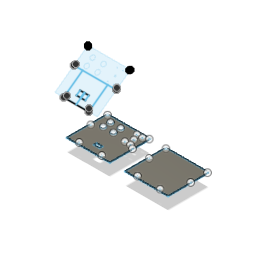
prop-blueprint (Autodesk Fusion 360 archive; units mm, degrees)
design "ledmatrix"
Autodesk Fusion 360 part; units mm, degrees
sketch "Sketch1" plane through (0, 0, 0) normal (0, 1, 0) x (1, 0, 0)
  line L0 (0, 0) -> (192, 0)
  line L1 (192, 0) -> (192, -96)
  line L2 (192, -96) -> (0, -96)
  line L3 (0, -96) -> (0, 0)
  line L4 (0, 0) -> (12, 0)
  line L5 (0, 0) -> (0, -10)
  line L6 (0, -10) -> (20.9444, -10)
  line L7 (12, 0) -> (12, -10)
  circle A0 centre (12, -10) radius 1.5
  circle A1 centre (113.3925, -144.8414) radius 15
  line L8 (283.7254, -24.5165) -> (335.7254, -24.5165)
  line L9 (335.7254, -24.5165) -> (335.7254, -119.5165)
  line L10 (335.7254, -119.5165) -> (283.7254, -119.5165)
  line L11 (283.7254, -119.5165) -> (283.7254, -24.5165)
  line L12 (283.7254, -24.5165) -> (290.7254, -24.5165)
  line L13 (290.7254, -24.5165) -> (290.7254, -30.5165)
  circle A2 centre (290.7254, -30.5165) radius 2.5
  dimension "d1" = 192
  dimension "d2" = 96
  dimension "d3" = 12
  dimension "d4" = 10
  dimension "d5" = 3
  dimension "d6" = 30
  dimension "d7" = 52
  dimension "d8" = 95
  dimension "d9" = 7
  dimension "d10" = 6
  dimension "d11" = 5
  constraint horizontal L0
  constraint vertical L1
  constraint horizontal L2
  constraint vertical L3
  constraint coincident L0.start L3.end
  constraint perpendicular L3 L4
  constraint perpendicular L4 L5
  constraint perpendicular L3 L6
  constraint coincident L6 L7.end
  constraint perpendicular L6 L7
  constraint coincident L7.end A0.centre
  constraint horizontal L8
  constraint vertical L9
  constraint horizontal L10
  constraint vertical L11
  constraint perpendicular L11 L12
  constraint perpendicular L12 L13
  constraint coincident L13.end A2.centre
  measures "d1" distance of L0.start L0.end
  measures "d2" distance of L0.start L2.end
  measures "d3" distance of L0.start L4.end
  measures "d4" distance of L0.start L5.end
  measures "d5" diameter of A0
  measures "d6" diameter of A1
  measures "d7" distance of L8.start L8.end
  measures "d8" distance of L8.start L10.end
  measures "d9" distance of L8.start L12.end
  measures "d10" distance of L12.end L13.end
  measures "d11" diameter of A2
sketch "Sketch2" plane through (96, 0, 48) normal (0, 1, 0) x (1, 0, 0)
  line L0 (-96, -48) -> (96, -48)
  line L1 (96, -48) -> (96, -58)
  line L2 (96, -58) -> (-96, -58)
  line L3 (-96, -58) -> (-96, -48)
  line L4 (-96, -58) -> (-116, -58)
  line L5 (-116, -58) -> (-116, 48)
  line L6 (-116, 48) -> (-96, 48)
  line L7 (-96, 48) -> (-96, -58)
  line L8 (96, -58) -> (116, -58)
  line L9 (116, -58) -> (116, 48)
  line L10 (116, 48) -> (96, 48)
  line L11 (96, 48) -> (96, -58)
  line L12 (-116, 48) -> (116, 48)
  line L13 (116, 48) -> (116, 58)
  line L14 (116, 58) -> (-116, 58)
  line L15 (-116, 58) -> (-116, 48)
  line L16 (-96, 38) -> (96, 38)
  line L17 (-84, 48) -> (-84, -48)
  line L18 (-96, -48) -> (-96, -38)
  line L19 (-96, -38) -> (96, -38)
  line L20 (96, -48) -> (84, -48)
  line L21 (96, -48) -> (84, -48)
  line L22 (84, -48) -> (84, 48)
  dimension "d12" = 10
  dimension "d13" = 20
  dimension "d14" = 20
  dimension "d15" = 10
  dimension "d16" = 192
  dimension "d17" = 96
  constraint horizontal L0
  constraint vertical L1
  constraint horizontal L2
  constraint vertical L3
  constraint horizontal L4
  constraint vertical L5
  constraint horizontal L6
  constraint vertical L7
  constraint horizontal L8
  constraint vertical L9
  constraint horizontal L10
  constraint vertical L11
  constraint horizontal L12
  constraint vertical L13
  constraint horizontal L14
  constraint vertical L15
  constraint coincident L7 L16.start
  constraint coincident L11 L16.end
  constraint perpendicular L11 L16
  constraint coincident L12 L17.start
  constraint coincident L0 L17.end
  constraint perpendicular L0 L17
  constraint coincident L7 L18.end
  constraint coincident L11 L19.end
  constraint perpendicular L11 L19
  constraint coincident L0 L20.end
  constraint coincident L12 L22.end
  constraint perpendicular L12 L22
  measures "d12" distance of L0.start L2.end
  measures "d13" distance of L2.end L4.end
  measures "d14" distance of L1.end L8.end
  measures "d15" distance of L5.end L14.end
  measures "d16" distance of L18.end L19.end
  measures "d17" distance of L17.start L17.end
extrude "Extrude1" add sketch "Sketch2" along normal blind 10 contours L0 L1 L2 L3 L7 L11 L20 L21 | L3 L4 L5 L6 L7 L12 L18 | L1 L8 L9 L10 L11 L12 | L6 L10 L12 L13 L14 L15 makes body 1
extrude "Extrude2" add sketch "Sketch2" against normal blind 10 contours L0 L7 L17 L18 L19 | L0 L1 L2 L3 L7 L11 L20 L21 | L3 L4 L5 L6 L7 L12 L18 | L0 L17 L19 L22 | L7 L16 L17 L19 | L0 L11 L19 L20 L21 L22 | L1 L8 L9 L10 L11 L12 | L7 L12 L16 L17 | L11 L16 L19 L22 | L12 L16 L17 L22 | L6 L10 L12 L13 L14 L15 | L11 L12 L16 L22 bodies 1
move_body "Move1" bodies 1 to x (1, 0, 0) y (0, 1, 0) z (0, 0, 1) at (260, 0, 0)
sketch "Sketch3" plane through (0, 0, 0) normal (0, 1, 0) x (1, 0, 0)
  line L0 (0, 0) -> (0, 136)
  line L1 (0, 0) -> (64.6952, 47.0588)
  line L2 (64.6952, 47.0588) -> (0, 136)
  dimension "d22" = 136
  dimension "d23" = 80
  constraint vertical L0
  measures "d22" distance of L0.start L0.end
  measures "d23" distance of L0.start L1.end
sketch "Sketch4" plane through (240, 0, 0) normal (-1, 0, 0) x (0, 0, 1)
  line L0 (106, -10) -> (106, 10)
  line L1 (106, 10) -> (-10, 10)
  line L2 (-10, 10) -> (-10, -10)
  line L3 (-10, -10) -> (106, -10)
  line L4 (-50, 10) -> (70.9677, -78.695)
  line L5 (70.9677, -78.695) -> (80.0728, -85.371)
  line L6 (150, 10) -> (80.0728, -85.371)
  line L7 (150, 10) -> (-50, 10)
  dimension "d27" = 150
  constraint perpendicular L5 L6
  constraint parallel L1 L7
  measures "d27" distance of L4.start L4.end
extrude "Extrude4" add sketch "Sketch4" along normal blind 30 separate body makes body 2
sketch "Sketch5" plane through (502, 0, 0) normal (1, 0, 0) x (0, 0, -1)
  line L0 (-80.0728, -85.371) -> (50, 10)
  line L1 (50, 10) -> (-150, 10)
  line L2 (-80.0728, -85.371) -> (-77.1163, -89.4032)
  line L3 (149.7307, 76.9238) -> (146.7742, 80.956)
  line L4 (-150, 10) -> (-80.0728, -85.371)
  line L5 (-80.0728, -85.371) -> (146.7742, 80.956)
  line L6 (149.7307, 76.9238) -> (-77.1163, -89.4032)
  dimension "d58" = 5
  constraint coincident L0.start L2.start
  constraint perpendicular L3 L5
  constraint perpendicular L2 L6
  measures "d58" distance of L3.end L3.start
move_body "Move6" bodies 1 to x (1, 0, 0) y (0, 1, 0) z (0, 0, 1) at (0, 0, -2.5)
sketch "Sketch6" plane through (472, 0, 0) normal (1, 0, 0) x (0, 0, -1)
  line L0 (12.5, -10) -> (12.5, 10)
  line L1 (12.5, 10) -> (-103.5, 10)
  line L2 (-103.5, 10) -> (-103.5, -10)
  line L3 (-103.5, -10) -> (12.5, -10)
  line L4 (12.5, -10) -> (40, 10)
  line L5 (40, 10) -> (12.5, 10)
  constraint coincident L0.start L3.end
  constraint coincident L0.end L1.start
  constraint perpendicular L0 L5
extrude "Extrude6" add sketch "Sketch6" against normal blind 232 contours L0 L4 L5 bodies 1
sketch "Sketch7" plane through (0, -17.3391, -12.7132) normal (0, 0.806452, 0.5913) x (1, 0, 0)
  line L0 (502, -115.0547) -> (502, 166.2356)
  line L1 (502, 166.2356) -> (210, 166.2356)
  line L2 (210, 166.2356) -> (210, -115.0547)
  line L3 (210, -115.0547) -> (502, -115.0547)
  line L4 (270, -103.7625) -> (270, -90)
  line L5 (270, -90) -> (270, 46)
  line L6 (240, 46) -> (240, -103.7625)
  line L7 (240, 46) -> (240, 46.2347)
  line L8 (240, 46.2347) -> (270, 46.2347)
  line L9 (270, 46.2347) -> (270, 46)
  line L10 (240, -103.7625) -> (240, -115.0547)
  line L11 (270, -103.7625) -> (270, -115.0547)
  line L12 (240, -115.0547) -> (270, -115.0547)
  dimension "d40" = 30
  constraint perpendicular L7 L8
  constraint coincident L3 L10.end
  constraint perpendicular L3 L10
  constraint coincident L3 L11.end
  constraint perpendicular L3 L11
  measures "d40" distance of L6.end L4.start
extrude "Extrude7" add sketch "Sketch7" along normal blind 10 contours L3 L4 L5 L6 L7 L8 L9 L10 L11 L12 bodies 2
sketch "Sketch8" plane through (240, 0, 0) normal (-1, 0, 0) x (0, 0, 1)
  line L0 (-49.7079, 10) -> (-33.0881, 10)
  line L1 (-33.0881, 10) -> (-43.897, 17.9252)
  line L2 (-49.7079, 10) -> (-33.0881, 10)
  line L3 (-33.0881, 19.9922) -> (-49.7079, 19.9922)
  line L4 (-33.0881, 19.9922) -> (-33.0881, 10)
  line L5 (-43.897, 17.9252) -> (-49.7079, 10)
  line L6 (-49.7079, 10) -> (-50, 10)
  line L7 (-50, 10) -> (-50, 20)
  line L8 (-50, 20) -> (-49.7079, 19.9922)
  constraint coincident L0.start L2.start
  constraint coincident L0.end L1.start
  constraint parallel L0 L3
  constraint perpendicular L3 L4
  constraint perpendicular L2 L7
extrude "Extrude8" cut sketch "Sketch8" against normal blind 30 bodies 2
sketch "Sketch9" plane through (240, 0, 0) normal (1, 0, 0) x (0, 0, -1)
  line L0 (-85.9858, -77.3065) -> (33.0881, 10)
  line L1 (33.0881, 10) -> (-150, 10)
  line L2 (33.0881, 10) -> (33.0881, 0)
  line L3 (33.0881, 0) -> (3.0881, 0)
  line L4 (33.0881, 10) -> (3.0881, 10)
  line L5 (-150, 10) -> (-85.9858, -77.3065)
  line L6 (3.0881, 0) -> (-11.9119, 0)
  line L7 (3.0881, 10) -> (-11.9119, 0)
  dimension "d45" = 30
  dimension "d98" = 30
  dimension "d99" = 15
  constraint coincident L0.end L1.start
  constraint perpendicular L1 L2
  constraint perpendicular L2 L3
  constraint coincident L1 L4.end
  constraint parallel L3 L6
  measures "d45" distance of L2.end L3.end
  measures "d98" distance of L0.end L4.end
  measures "d99" distance of L3.end L6.end
extrude "Extrude9" add sketch "Sketch9" along normal blind 30 contours L0 L1 L3 L4 L6 L7 bodies 2
move_body "Move7" bodies 1 to x (1, 0, 0) y (0, 1, 0) z (0, 0, 1) at (0, -5, 15)
move_body "Move8" bodies 1 to x (1, 0, 0) y (0, 1, 0) z (0, 0, 1) at (0, -5, 6)
move_body "Move9" bodies 1 to x (1, 0, 0) y (0, 1, 0) z (0, 0, 1) at (0, 0, -0.5)
move_body "Move10" bodies 1 to x (1, 0, 0) y (0, 1, 0) z (0, 0, 1) at (0, 0, -0.1)
sketch "Sketch10" plane through (240, 0, 0) normal (1, 0, 0) x (0, 0, -1)
  line L0 (3.0881, 10) -> (-150, 10)
  line L1 (-150, 10) -> (-85.9858, -77.3065)
  line L2 (-85.9858, -77.3065) -> (19.4495, 0)
  line L3 (19.4495, 0) -> (-11.9119, 0)
  line L4 (-8.25, -20) -> (-8.25, -20.3096)
  line L5 (-8.25, -20.3096) -> (-68.25, -20.3096)
  line L6 (-68.25, -20.3096) -> (-68.25, -30.3096)
  line L7 (-8.25, -20.3096) -> (-21.8886, -30.3096)
  line L8 (-68.25, -30.3096) -> (-52.0404, -52.4173)
  line L9 (-124, 0) -> (-109, 0)
  line L10 (-109, 0) -> (-109, 10)
  line L11 (-109, 10) -> (-124, 10)
  line L12 (-124, 10) -> (-124, 0)
  line L13 (-11.9119, 0) -> (3.0881, 10)
  dimension "d50" = 10
  dimension "d51" = 60
  dimension "d91" = 15
  constraint coincident L2 L4.end
  constraint vertical L4
  constraint perpendicular L4 L5
  constraint perpendicular L5 L6
  constraint coincident L2 L7.end
  constraint coincident L2 L8.end
  constraint perpendicular L2 L8
  constraint horizontal L9
  constraint vertical L10
  constraint horizontal L11
  constraint vertical L12
  measures "d50" distance of L5.end L6.end
  measures "d51" distance of L4.end L5.end
  measures "d91" distance of L9.start L9.end
extrude "Extrude18" add sketch "Sketch10" along normal blind 30 contours L2 L5 L6 L7 L8 bodies 2
mirror "Mirror1" about plane through (0, 0, 0) normal (1, 0, 0) of bodies 2 makes body 3
sketch "Sketch11" plane through (0, -17.3391, -12.7132) normal (0, 0.806452, 0.5913) x (1, 0, 0)
  line L0 (502, -115.0547) -> (502, 166.2356)
  line L1 (502, 166.2356) -> (210, 166.2356)
  line L2 (210, 166.2356) -> (210, -115.0547)
  line L3 (210, -115.0547) -> (502, -115.0547)
  line L4 (475, 150) -> (423, 150)
  line L5 (423, 150) -> (423, 55)
  line L6 (423, 55) -> (475, 55)
  line L7 (475, 55) -> (475, 150)
  line L8 (423, 150) -> (430, 150)
  line L9 (430, 150) -> (430, 144)
  circle A0 centre (430, 144) radius 2.5
  line L10 (475, 150) -> (468, 150)
  line L11 (468, 150) -> (468, 144)
  circle A1 centre (468, 144) radius 2.5
  line L12 (475, 55) -> (468, 55)
  line L13 (468, 55) -> (468, 61)
  circle A2 centre (468, 61) radius 2.5
  line L14 (423, 55) -> (430, 55)
  line L15 (430, 55) -> (430, 61)
  circle A3 centre (430, 61) radius 2.5
  line L16 (423, 150) -> (449, 150)
  line L17 (449, 55) -> (449, 150)
  line L18 (475, 150) -> (475, 102.5)
  line L19 (475, 102.5) -> (423, 102.5)
  circle A4 centre (449, 102.5) radius 5
  dimension "d59" = 52
  dimension "d60" = 95
  dimension "d61" = 6
  dimension "d62" = 5
  dimension "d63" = 7
  dimension "d64" = 6
  dimension "d65" = 5
  dimension "d66" = 7
  dimension "d67" = 6
  dimension "d68" = 5
  dimension "d69" = 7
  dimension "d70" = 6
  dimension "d71" = 5
  dimension "d80" = 10
  constraint horizontal L4
  constraint vertical L5
  constraint horizontal L6
  constraint vertical L7
  constraint coincident L4 L8.end
  constraint perpendicular L4 L9
  constraint coincident L9.end A0.centre
  constraint perpendicular L7 L10
  constraint perpendicular L4 L11
  constraint coincident L11.end A1.centre
  constraint perpendicular L7 L12
  constraint perpendicular L12 L13
  constraint coincident L13.end A2.centre
  constraint perpendicular L5 L14
  constraint perpendicular L14 L15
  constraint coincident L15.end A3.centre
  constraint midpoint L4 L16.end
  constraint midpoint L6 L17.start
  constraint midpoint L7 L18.end
  constraint midpoint L5 L19.end
  constraint midpoint L19 A4.centre
  measures "d59" distance of L4.start L4.end
  measures "d60" distance of L4.start L6.end
  measures "d61" distance of L8.end L9.end
  measures "d62" diameter of A0
  measures "d63" distance of L4.start L10.end
  measures "d64" distance of L10.end L11.end
  measures "d65" diameter of A1
  measures "d66" distance of L6.end L12.end
  measures "d67" distance of L12.end L13.end
  measures "d68" diameter of A2
  measures "d69" distance of L5.end L14.end
  measures "d70" distance of L14.end L15.end
  measures "d71" diameter of A3
  measures "d80" diameter of A4
sketch "Sketch12" plane through (0, -17.3391, -12.7132) normal (0, 0.806452, 0.5913) x (1, 0, 0)
  circle A0 centre (275, 125) radius 15
  circle A1 centre (350, 125) radius 15
  circle A2 centre (275, 75) radius 15
  circle A3 centre (350, 75) radius 15
  dimension "d72" = 30
  dimension "d73" = 30
  dimension "d74" = 30
  dimension "d75" = 30
  measures "d72" diameter of A0
  measures "d73" diameter of A1
  measures "d74" diameter of A2
  measures "d75" diameter of A3
sketch "Sketch13" plane through (0, -21.3714, -15.6697) normal (0, -0.806452, -0.5913) x (-1, 0, 0)
  circle A0 centre (-430, 61) radius 2.5
  circle A1 centre (-468, 144) radius 2.5
  circle A2 centre (-468, 61) radius 2.5
  circle A3 centre (-430, 144) radius 2.5
  circle A4 centre (-449, 102.5) radius 5
  circle A5 centre (-350, 75) radius 15
  circle A6 centre (-350, 125) radius 15
  circle A7 centre (-275, 75) radius 15
  circle A8 centre (-275, 125) radius 15
  line L0 (-502, 166.2356) -> (-502, -115.0547)
  line L1 (-502, -115.0547) -> (-210, -115.0547)
  line L2 (-210, -115.0547) -> (-210, 166.2356)
  line L3 (-210, 166.2356) -> (-502, 166.2356)
  line L4 (-335, 125) -> (-290, 125)
  line L5 (-350, 110) -> (-350, 90)
  line L6 (-275, 110) -> (-275, 90)
  line L7 (-335, 75) -> (-290, 75)
  line L8 (-350, 100) -> (-275, 100)
  line L9 (-350, 100) -> (-361, 100)
  line L10 (-350, 100) -> (-355, 100)
  line L11 (-355, 100) -> (-355, 110.8579)
  line L12 (-350, 100) -> (-345, 100)
  line L13 (-345, 100) -> (-345, 110.8579)
  line L14 (-345, 100) -> (-345, 89.1421)
  line L15 (-355, 100) -> (-355, 89.1421)
  line L16 (-275, 100) -> (-270, 100)
  line L17 (-270, 100) -> (-270, 89.1421)
  line L18 (-270, 100) -> (-270, 110.8579)
  line L19 (-275, 100) -> (-280, 100)
  line L20 (-280, 100) -> (-280, 110.8579)
  line L21 (-280, 100) -> (-280, 89.1421)
  line L22 (-355, 89.1421) -> (-355, -115.0547)
  line L23 (-345, 89.1421) -> (-345, 80)
  line L24 (-345, 80) -> (-345, -115.0547)
  line L25 (-280, 89.1421) -> (-280, -115.0547)
  line L26 (-270, 89.1421) -> (-270, -115.0547)
  line L27 (-355, -115.0547) -> (-345, -115.0547)
  line L28 (-280, -115.0547) -> (-270, -115.0547)
  line L29 (-355, 110.8579) -> (-350, 110)
  line L30 (-345, 110.8579) -> (-350, 110)
  line L31 (-280, 110.8579) -> (-275, 110)
  line L32 (-270, 110.8579) -> (-275, 110)
  dimension "d81" = 5
  dimension "d82" = 5
  dimension "d83" = 10.8579
  constraint coincident A6 L4.start
  constraint coincident A8 L4.end
  constraint parallel L3 L4
  constraint coincident A6 L5.start
  constraint coincident A5 L5.end
  constraint perpendicular L4 L5
  constraint coincident A8 L6.start
  constraint coincident A7 L6.end
  constraint parallel L5 L6
  constraint coincident A5 L7.start
  constraint coincident A7 L7.end
  constraint perpendicular L6 L7
  constraint midpoint L5 L8.start
  constraint midpoint L6 L8.end
  constraint perpendicular L5 L9
  constraint coincident L9 L10.end
  constraint perpendicular L5 L10
  constraint coincident A6 L11.end
  constraint perpendicular L10 L11
  constraint coincident L8 L12.end
  constraint perpendicular L5 L12
  constraint coincident A6 L13.end
  constraint perpendicular L8 L13
  constraint coincident A5 L14.end
  constraint perpendicular L8 L14
  constraint coincident A5 L15.end
  constraint perpendicular L10 L15
  constraint perpendicular L6 L16
  constraint coincident A7 L17.end
  constraint perpendicular L8 L17
  constraint coincident A8 L18.end
  constraint perpendicular L16 L18
  constraint coincident L8 L19.end
  constraint perpendicular L6 L19
  constraint coincident A8 L20.end
  constraint perpendicular L19 L20
  constraint coincident A7 L21.end
  constraint perpendicular L8 L21
  constraint coincident L1 L22.end
  constraint perpendicular L1 L22
  constraint coincident L1 L24.end
  constraint perpendicular L1 L24
  constraint coincident L1 L25.end
  constraint perpendicular L1 L25
  constraint coincident L1 L26.end
  constraint perpendicular L1 L26
  measures "d81" distance of L8.end L19.end
  measures "d82" distance of L8.start L12.end
  measures "d83" distance of L12.end L13.end
extrude "Extrude15" cut 1 faces at (264, -10, 78.5667) along direction (0, -1, 0) blind 3 on bodies 1 bodies 1
fillet "Fillet1" radius 7.5 2 edges at (225, 10, 150) (-225, 10, 150) on bodies 2 3
move_body "Move15" bodies 3 to x (1, 0, 0) y (0, 1, 0) z (0, 0, 1) at (162, 0, 0)
sketch "Sketch15" plane through (0, -17.3391, -12.7132) normal (0, 0.806452, 0.5913) x (1, 0, 0)
  circle A0 centre (55, 61) radius 2.5
  circle A1 centre (93, 144) radius 2.5
  circle A2 centre (93, 61) radius 2.5
  circle A3 centre (55, 144) radius 2.5
  circle A4 centre (74, 102.5) radius 5
  circle A5 centre (-25, 75) radius 15
  circle A6 centre (-25, 125) radius 15
  circle A7 centre (-100, 75) radius 15
  circle A8 centre (-100, 125) radius 15
  line L0 (127, -115.0547) -> (127, 166.2356)
  line L1 (127, 166.2356) -> (-165, 166.2356)
  line L2 (-165, 166.2356) -> (-165, -115.0547)
  line L3 (-165, -115.0547) -> (127, -115.0547)
  line L4 (-165, 166.2356) -> (-160, 166.2356)
  line L5 (-160, 166.2356) -> (-160, 161.2356)
  line L6 (-160, 161.2356) -> (-165, 161.2356)
  line L7 (-165, 161.2356) -> (-165, 166.2356)
  circle A9 centre (-160, 161.2356) radius 1.5
  line L8 (127, 166.2356) -> (122, 166.2356)
  line L9 (122, 166.2356) -> (122, 161.2356)
  line L10 (122, 161.2356) -> (127, 161.2356)
  line L11 (127, 161.2356) -> (127, 166.2356)
  circle A10 centre (122, 161.2356) radius 1.5
  line L12 (-165, 46.3093) -> (-160, 46.3093)
  line L13 (-160, 46.3093) -> (-160, 56.3093)
  line L14 (-160, 56.3093) -> (-165, 56.3093)
  line L15 (-165, 56.3093) -> (-165, 46.3093)
  circle A11 centre (-160, 56.3093) radius 1.5
  line L16 (-160, 46.3093) -> (127, 46.3093)
  line L17 (127, 46.3093) -> (122, 46.3093)
  line L18 (122, 46.3093) -> (122, 56.3093)
  line L19 (122, 56.3093) -> (127, 56.3093)
  line L20 (127, 56.3093) -> (127, 46.3093)
  circle A12 centre (122, 56.3093) radius 1.5
  line L21 (-104.9331, 46.3093) -> (-104.9331, -115.0547)
  line L22 (67.0003, 46.3093) -> (67.0003, -115.0547)
  line L23 (67.0003, -115.0547) -> (57.0003, -115.0547)
  line L24 (57.0003, -115.0547) -> (57.0003, -100.0547)
  line L25 (57.0003, -100.0547) -> (67.0003, -100.0547)
  line L26 (67.0003, -100.0547) -> (67.0003, -115.0547)
  line L27 (-104.9331, -115.0547) -> (-94.9331, -115.0547)
  line L28 (-94.9331, -115.0547) -> (-94.9331, -100.0547)
  line L29 (-94.9331, -100.0547) -> (-104.9331, -100.0547)
  line L30 (-104.9331, -100.0547) -> (-104.9331, -115.0547)
  circle A13 centre (-94.9331, -100.0547) radius 1.5
  circle A14 centre (57.0003, -100.0547) radius 1.5
  line L31 (-104.9331, -115.0547) -> (67.0003, -115.0547)
  line L32 (-18.9664, -115.0547) -> (-18.9664, -45.0547)
  line L33 (-18.9664, -45.0547) -> (11.0336, -45.0547)
  line L34 (11.0336, -45.0547) -> (11.0336, -75.0547)
  line L35 (11.0336, -75.0547) -> (-18.9664, -75.0547)
  line L36 (-18.9664, -75.0547) -> (-18.9664, -45.0547)
  line L37 (-18.9664, -45.0547) -> (-48.9664, -45.0547)
  line L38 (-48.9664, -45.0547) -> (-48.9664, -75.0547)
  line L39 (-48.9664, -75.0547) -> (-18.9664, -75.0547)
  line L40 (-18.9664, -75.0547) -> (-18.9664, -45.0547)
  dimension "d100" = 5
  dimension "d101" = 5
  dimension "d102" = 3
  dimension "d103" = 5
  dimension "d104" = 5
  dimension "d105" = 3
  dimension "d106" = 5
  dimension "d107" = 10
  dimension "d108" = 3
  dimension "d109" = 5
  dimension "d110" = 10
  dimension "d111" = 3
  dimension "d112" = 10
  dimension "d113" = 15
  dimension "d114" = 10
  dimension "d115" = 15
  dimension "d116" = 3
  dimension "d117" = 3
  dimension "d118" = 171.9334
  dimension "d120" = 70
  dimension "d121" = 30
  dimension "d122" = 30
  dimension "d123" = 30
  dimension "d124" = 30
  constraint horizontal L4
  constraint vertical L5
  constraint horizontal L6
  constraint vertical L7
  constraint coincident L1.end L2.start
  constraint coincident L5.end L6.start
  constraint horizontal L8
  constraint vertical L9
  constraint horizontal L10
  constraint vertical L11
  constraint coincident L0.end L1.start
  constraint coincident L9.end L10.start
  constraint horizontal L12
  constraint vertical L13
  constraint horizontal L14
  constraint vertical L15
  constraint coincident L2 L12.start
  constraint coincident L13.end L14.start
  constraint coincident L0 L16.end
  constraint perpendicular L0 L16
  constraint horizontal L17
  constraint vertical L18
  constraint horizontal L19
  constraint vertical L20
  constraint coincident L18.end L19.start
  constraint coincident L16 L21.start
  constraint coincident L3 L21.end
  constraint perpendicular L3 L21
  constraint coincident L16 L22.start
  constraint coincident L3 L22.end
  constraint perpendicular L3 L22
  constraint horizontal L23
  constraint vertical L24
  constraint horizontal L25
  constraint vertical L26
  constraint horizontal L27
  constraint vertical L28
  constraint horizontal L29
  constraint vertical L30
  constraint coincident L28.end L29.start
  constraint coincident L24.end L25.start
  constraint perpendicular L26 L31
  constraint midpoint L31 L32.start
  constraint perpendicular L31 L32
  constraint horizontal L33
  constraint vertical L34
  constraint horizontal L35
  constraint vertical L36
  constraint horizontal L37
  constraint vertical L38
  constraint horizontal L39
  constraint vertical L40
  measures "d100" distance of L1.end L4.end
  measures "d101" distance of L1.end L6.end
  measures "d102" diameter of A9
  measures "d103" distance of L0.end L8.end
  measures "d104" distance of L0.end L10.end
  measures "d105" diameter of A10
  measures "d106" distance of L12.start L12.end
  measures "d107" distance of L12.start L14.end
  measures "d108" diameter of A11
  measures "d109" distance of L16.end L17.end
  measures "d110" distance of L16.end L19.end
  measures "d111" diameter of A12
  measures "d112" distance of L22.end L23.end
  measures "d113" distance of L22.end L25.end
  measures "d114" distance of L21.end L27.end
  measures "d115" distance of L21.end L29.end
  measures "d116" diameter of A13
  measures "d117" diameter of A14
  measures "d118" distance of L21.end L22.end
  measures "d120" distance of L32.start L32.end
  measures "d121" distance of L32.end L33.end
  measures "d122" distance of L32.end L35.end
  measures "d123" distance of L32.end L37.end
  measures "d124" distance of L32.end L35.end
sketch "Sketch16" plane through (0, -17.3391, -12.7132) normal (0, 0.806452, 0.5913) x (1, 0, 0)
  circle A0 centre (122, 161.2356) radius 1.5
  line L0 (-48.9664, -75.0547) -> (-48.9664, -45.0547)
  line L1 (-48.9664, -45.0547) -> (11.0336, -45.0547)
  line L2 (11.0336, -45.0547) -> (11.0336, -75.0547)
  line L3 (11.0336, -75.0547) -> (-48.9664, -75.0547)
  circle A1 centre (122, 56.3093) radius 1.5
  circle A2 centre (-160, 161.2356) radius 1.5
  circle A3 centre (-94.9331, -100.0547) radius 1.5
  circle A4 centre (57.0003, -100.0547) radius 1.5
  circle A5 centre (-160, 56.3093) radius 1.5
  circle A6 centre (55, 61) radius 2.5
  circle A7 centre (93, 144) radius 2.5
  circle A8 centre (93, 61) radius 2.5
  circle A9 centre (55, 144) radius 2.5
  circle A10 centre (74, 102.5) radius 5
  circle A11 centre (-25, 75) radius 15
  circle A12 centre (-25, 125) radius 15
  circle A13 centre (-100, 75) radius 15
  circle A14 centre (-100, 125) radius 15
  line L4 (127, -115.0547) -> (127, 166.2356)
  line L5 (127, 166.2356) -> (-165, 166.2356)
  line L6 (-165, 166.2356) -> (-165, -115.0547)
  line L7 (-165, -115.0547) -> (127, -115.0547)
sketch "Sketch17" plane through (0, 0, 0) normal (0, 1, 0) x (1, 0, 0)
  line L0 (367.0049, -345.3696) -> (367.0046, -325.2726)
  circle A0 centre (362.0004, -205.3796) radius 15
  circle A1 centre (362.0004, -155.3796) radius 15
  line L1 (407.0046, -325.2908) -> (407, -345.2908)
  circle A2 centre (474, -177.1591) radius 5
  line L2 (407, -345.2908) -> (367.0049, -345.3696)
  line L3 (367.0046, -325.2726) -> (407.0046, -325.2908)
  circle A3 centre (522, -120.0645) radius 1.5
  line L4 (527, -395.0547) -> (527, -115.0547)
  circle A4 centre (302.0006, -380.4976) radius 1.5
  circle A5 centre (457.0003, -380.1925) radius 1.5
  line L5 (232.0006, -395.6355) -> (527, -395.0547)
  circle A6 centre (522, -235.0647) radius 1.5
  circle A7 centre (454, -136) radius 2.5
  circle A8 centre (292.0006, -205.5174) radius 15
  circle A9 centre (492, -219) radius 2.5
  circle A10 centre (492, -136) radius 2.5
  circle A11 centre (454, -219) radius 2.5
  circle A12 centre (292.0006, -155.5174) radius 15
  circle A13 centre (237.0006, -235.6259) radius 1.5
  line L6 (232.0006, -115.6355) -> (232.0006, -395.6355)
  circle A14 centre (237.0006, -120.6257) radius 1.5
  line L7 (527, -115.0547) -> (232.0006, -115.6355)
  line L8 (927, -395.0547) -> (927, -115.0547)
  circle A15 centre (922, -235.0547) radius 1.5
  line L9 (927, -115.0547) -> (632, -115.0547)
  circle A16 centre (857.0003, -380.0547) radius 1.5
  circle A17 centre (702, -380.0547) radius 1.5
  line L10 (632, -395.0547) -> (927, -395.0547)
  circle A18 centre (637, -235.0547) radius 1.5
  circle A19 centre (637, -120.0547) radius 1.5
  circle A20 centre (922, -120.0547) radius 1.5
  line L11 (632, -115.0547) -> (632, -395.0547)
  dimension "d138" = 280
  dimension "d139" = 295
  dimension "d140" = 5
  dimension "d141" = 3
  dimension "d142" = 5
  dimension "d143" = 40
  dimension "d144" = 60
  dimension "d145" = 40
  dimension "d146" = 70
  dimension "d147" = 50
  dimension "d148" = 60
  dimension "d149" = 50
  dimension "d150" = 70
  dimension "d151" = 5
  dimension "d152" = 5
  dimension "d153" = 35
  dimension "d155" = 38
  dimension "d156" = 38
  dimension "d157" = 35
  dimension "d158" = 83
  dimension "d159" = 83
  dimension "d160" = 62
  dimension "d161" = 53
  dimension "d162" = 5
  dimension "d163" = 120
  dimension "d164" = 5
  dimension "d165" = 120
  dimension "d166" = 15
  dimension "d167" = 69.9997
  dimension "d168" = 70
  dimension "d169" = 15
  dimension "d170" = 20
  dimension "d171" = 40
  dimension "d172" = 50
  dimension "d173" = 120
  dimension "d174" = 280
  dimension "d175" = 295
  dimension "d176" = 5
  dimension "d177" = 3
  dimension "d178" = 5
  dimension "d187" = 5
  dimension "d188" = 5
  dimension "d197" = 5
  dimension "d198" = 120
  dimension "d199" = 5
  dimension "d200" = 120
  dimension "d201" = 15
  dimension "d202" = 69.9997
  dimension "d203" = 70
  dimension "d204" = 15
  dimension "d211" = 295
  dimension "d216" = 280
  measures "d138" distance of L4.start L4.end
  measures "d139" distance of L4.end L6.start
  measures "d140" distance of A14.centre L6
  measures "d141" diameter of A14
  measures "d142" distance of A14.centre L7
  measures "d143" distance of A12.centre L7
  measures "d144" distance of A12.centre L6
  measures "d145" distance of A1.centre L7
  measures "d146" distance of A12.centre A1.centre
  measures "d147" vertical distance of A12.centre A8.centre
  measures "d148" distance of A8.centre L6
  measures "d149" vertical distance of A1.centre A0.centre
  measures "d150" distance of A8.centre A0.centre
  measures "d151" distance of A3.centre L4
  measures "d152" distance of A3.centre L7
  measures "d153" distance of A10.centre L4
  measures "d155" distance of A9.centre A11.centre
  measures "d156" distance of A10.centre A7.centre
  measures "d157" distance of A9.centre L4
  measures "d158" distance of A10.centre A9.centre
  measures "d159" distance of A7.centre A11.centre
  measures "d160" distance of A2.centre L7
  measures "d161" distance of A2.centre L4
  measures "d162" distance of A13.centre L6
  measures "d163" distance of A13.centre L7
  measures "d164" distance of A6.centre L4
  measures "d165" distance of A6.centre L7
  measures "d166" distance of A5.centre L5
  measures "d167" distance of A5.centre L4
  measures "d168" distance of A4.centre L6
  measures "d169" distance of A4.centre L5
  measures "d170" distance of L1.start L1.end
  measures "d171" distance of L0.end L1.start
  measures "d172" distance of L2 L5
  measures "d173" distance of L1.end L4
  measures "d174" distance of L8.end L8.start
  measures "d175" distance of L8.end L9.end
  measures "d176" distance of A19.centre L11
  measures "d177" diameter of A19
  measures "d178" distance of A19.centre L9
  measures "d187" distance of A20.centre L8
  measures "d188" distance of A20.centre L9
  measures "d197" distance of A18.centre L11
  measures "d198" distance of A18.centre L9
  measures "d199" distance of A15.centre L8
  measures "d200" distance of A15.centre L9
  measures "d201" distance of A16.centre L10
  measures "d202" distance of A16.centre L8
  measures "d203" distance of A17.centre L11
  measures "d204" distance of A17.centre L10
  measures "d211" distance of L4.start L5.start
  measures "d216" vertical distance of L5.start L6.start
extrude "Extrude25" add sketch "Sketch17" along normal blind 3 separate body contours L4 L5 L6 L7 makes body 4
extrude "Extrude26" add sketch "Sketch17" along normal blind 3 separate body contours L8 L9 L10 L11 makes body 5
extrude "Extrude20" [suppressed]
extrude "Extrude21" [suppressed]
extrude "Extrude22" [suppressed]
extrude "Extrude23" [suppressed]
extrude "Extrude24" [suppressed]
copy_body "CopyPasteBodies3" [suppressed]
move_body "Move17" [suppressed]
move_body "Move18" [suppressed]
move_body "Move19" [suppressed]
hidden bodies 1 2 3
